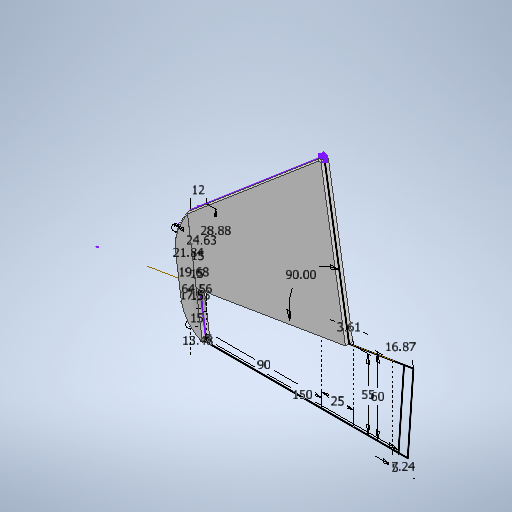
# Autodesk Inventor part: Part14
Saved by Autodesk Inventor 2025.3 (Build 293356000, 356)
## iProperties
Created: 2025-07-08
Part Number: Part14
Material: Generic
Document SubType Name: Modeling
Designer: steve
Density: 1 g/cm^3
Appearance: Default
Author: steve
Autodesk Inventor part; units mm, degrees
ref_plane "YZ Plane" through (0, 0, 0) normal (1, 0, 0) x (0, 1, 0)
ref_plane "XZ Plane" through (0, 0, 0) normal (0, 1, 0) x (-1, 0, 0)
ref_plane "XY Plane" through (0, 0, 0) normal (0, 0, 1) x (1, 0, 0)
sketch "Sketch1" plane through (0, 0, 0) normal (0, 0, 1) x (1, 0, 0)
  line L0 (0, 0) -> (150, 0)
  line L1 (150, 0) -> (157.24, 0)
  line L2 (0, 0) -> (0, 64.56) construction
  line L3 (0, 64.56) -> (0, 93.44) construction
  line L4 (0, 0) -> (0, 5)
  line L5 (0, 5) -> (-13.48, 5) construction
  line L6 (0, 5) -> (0, 20) construction
  line L7 (0, 20) -> (-17.53, 20) construction
  line L8 (0, 20) -> (0, 35) construction
  line L9 (0, 35) -> (-19.68, 35) construction
  line L10 (0, 35) -> (0, 50) construction
  line L11 (0, 50) -> (-21.84, 50) construction
  line L12 (0, 50) -> (0, 65) construction
  line L13 (0, 65) -> (-24.63, 65) construction
  line L14 (0, 0) -> (90, 0)
  line L15 (90, 0) -> (90, 169.8701) construction
  line L16 (90, 169.8701) -> (0, 93.44)
  line L17 (90, 169.8701) -> (92.1952, 169.8701)
  line L18 (90, 0) -> (115, 0)
  line L19 (115, 0) -> (115, 55) construction
  line L20 (115, 55) -> (111.4391, 54.4065)
  line L21 (150, 0) -> (145, 0)
  line L22 (145, 0) -> (145, 60) construction
  line L23 (145, 60) -> (161.6405, 62.7734)
  line L24 (157.24, 0) -> (161.6405, 62.7734)
  line L25 (145, 60) -> (115, 55)
  line L26 (111.4391, 54.4065) -> (92.1952, 169.8701)
  spline S0 degree 2 poles (90, 169.8701) (91.3956, 172.0746) (92.1952, 169.8701) knots 0 0 0 1 1 1
  line L27 (-12, -16.1926) -> (-12, 83.2493) construction
  line L28 (0, 93.44) -> (-12, 83.2493)
  line L29 (-12, 83.2493) -> (0, 0)
  line L30 (-21.84, 50) -> (-17.53, 20)
  line L31 (0, 0) -> (-13.48, 5) construction
  line L32 (-13.48, 5) -> (-17.53, 20) construction
  spline S1 degree 2 poles (0, 0) (-13.48, 5) (-17.53, 20) knots 1 1 1 2 2 2
  line L33 (-21.84, 50) -> (-24.63, 65) construction
  line L34 (-24.63, 65) -> (-12, 83.2493) construction
  spline S2 degree 2 poles (-21.84, 50) (-24.63, 65) (-12, 83.2493) knots 1 1 1 2 2 2
  line L35 (150, 0) -> (154.3149, 61.5525)
  line L36 (111.4391, 54.4065) -> (-5.044, 34.9927)
  line L37 (-84.3983, 21.7669) -> (-85.9636, 21.5061)
  line L38 (111.4391, 54.4065) -> (-2.1779, 35.4703)
  point P0 (91.2953, 170.9702)
  point P1 (-6, 88.3447)
  dimension "d0" = 150
  dimension "d1" = 7.24
  dimension "d2" = 64.56
  dimension "d3" = 28.88
  dimension "d4" = 13.48
  dimension "d5" = 15
  dimension "d6" = 17.53
  dimension "d7" = 15
  dimension "d8" = 19.68
  dimension "d9" = 15
  dimension "d10" = 21.84
  dimension "d11" = 15
  dimension "d12" = 24.63
  dimension "d14" = 90
  dimension "d17" = 25
  dimension "d18" = 55
  dimension "d19" = 3.61
  dimension "d20" = 5
  dimension "d21" = 60
  dimension "d22" = 16.87
  dimension "d24" = 12
  dimension "d25" = 5
  dimension "d49" = 90
  constraints: 70 end point, 17 point on line, 9 perpendicular, 5 collinear, 2 coincident, 2 vertical, 1 horizontal, 1 midpoint, 1 parallel, 9 other
  measures "d0" distance of L0.start L0.end
  measures "d1" distance of L0.end L1.end
  measures "d2" distance of L0.start L2.end
  measures "d3" distance of L2.end L3.end
  measures "d4" distance of L4.end L5.end
  measures "d5" distance of L4.end L6.end
  measures "d6" distance of L6.end L7.end
  measures "d7" distance of L6.end L8.end
  measures "d8" distance of L8.end L9.end
  measures "d9" distance of L8.end L10.end
  measures "d10" distance of L10.end L11.end
  measures "d11" distance of L10.end L12.end
  measures "d12" distance of L12.end L13.end
  measures "d14" distance of L0.start L14.end
  measures "d17" distance of L14.end L18.end
  measures "d18" distance of L18.end L19.end
  measures "d19" distance of L19.end L20.end
  measures "d20" distance of L0.end L21.end
  measures "d21" distance of L21.end L22.end
  measures "d22" distance of L23.end L22.end
  measures "d24" distance between parallel lines of L27 L3
  measures "d25" distance of L0.start L4.end
  measures "d49" angle of L38 L26
extrude "Extrusion1" add sketch "Sketch1" along normal mid plane 5.8 contours S1 L30 S2 L29
extrude "Extrusion2" add sketch "Sketch1" along normal mid plane 5.7 contours L29 L28 L16 L17 L26 L36
fillet "Fillet2" radius 1 4 edges at (91.0976, 169.8701, 2.85) (39, 126.5597, 2.85) (39, 126.5597, -2.85) (91.0976, 169.8701, -2.85)
fillet "Fillet3" radius 1 6 edges at (-20.775, 65.8123, 2.9) (-20.775, 65.8123, -2.9) (-19.685, 35, 2.9) (-11.1225, 7.5, 2.9) (-19.685, 35, -2.9) (-11.1225, 7.5, -2.9)
sketch "Sketch2" plane through (-5.044, 34.9927, 2.85) normal (0.9897702, 0.1426708, 0) x (0, 0, -1)
  line L0 (5.7, 0) -> (0, 0) projected
  circle A0 centre (2.85, 0) radius 1.5
  point P0 (2.85, -35.3543)
  dimension "d45" = 3
  constraints: 1 centre point, 1 coincident, 1 midpoint
  measures "d45" diameter of A0
extrude "Extrusion6" cut sketch "Sketch2" against normal blind 2
body "Solid1"
